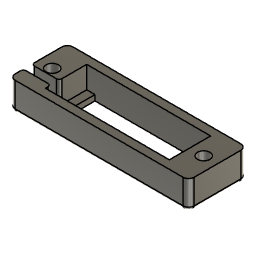
BracketLD2450 (Autodesk Fusion 360 design; units mm, degrees)
Autodesk Fusion 360 part; units mm, degrees
note: some values were not read from the file. Set by a fixed rule: the direction of a hole.
sketch "Sketch1" plane through (0, 0, 0) normal (0, 0, 1) x (1, 0, 0)
  line L0 (0, 0) -> (45, 0)
  line L1 (45, 0) -> (45, 15)
  line L2 (45, 15) -> (0, 15)
  line L3 (0, 15) -> (0, 0)
  line L4 (-10, -3) -> (55, -3)
  line L5 (55, -3) -> (55, 18)
  line L6 (55, 18) -> (-10, 18)
  line L7 (-10, 18) -> (-10, -3)
  line L8 (0, 7.5) -> (-5, 7.5)
  line L9 (45, 7.5) -> (50, 7.5)
  line L10 (0, 15) -> (3, 15)
  line L11 (3, 15) -> (3, 0)
  line L12 (3, 0) -> (0, 0)
  line L13 (0, 0) -> (0, 15)
  line L14 (45, 15) -> (42, 15)
  line L15 (42, 15) -> (42, 0)
  line L16 (42, 0) -> (45, 0)
  line L17 (45, 0) -> (45, 15)
  line L18 (0, 0) -> (0, 2)
  line L19 (0, 2) -> (-10, 2)
  line L20 (-10, 2) -> (-10, 5)
  line L21 (-10, 5) -> (0, 5)
  line L22 (0, 5) -> (0, 2)
  dimension "d1" = 45
  dimension "d2" = 15
  dimension "d5" = 65
  dimension "d6" = 21
  dimension "d7" = 5
  dimension "d8" = 5
  dimension "d9" = 3
  dimension "d10" = 15
  dimension "d11" = 3
  dimension "d19" = 2
  dimension "d20" = 3
  constraint horizontal L0
  constraint vertical L1
  constraint horizontal L2
  constraint vertical L3
  constraint coincident L0.start L3.end
  constraint horizontal L4
  constraint vertical L5
  constraint horizontal L6
  constraint vertical L7
  constraint midpoint L3 L8.start
  constraint perpendicular L7 L8
  constraint midpoint L1 L9.start
  constraint perpendicular L1 L9
  constraint horizontal L10
  constraint vertical L11
  constraint horizontal L12
  constraint vertical L13
  constraint horizontal L14
  constraint vertical L15
  constraint horizontal L16
  constraint vertical L17
  constraint perpendicular L12 L18
  constraint horizontal L19
  constraint vertical L20
  constraint horizontal L21
  constraint vertical L22
  measures "d1" distance of L0.start L0.end
  measures "d2" distance of L0.start L2.end
  measures "d5" distance of L4.start L4.end
  measures "d6" distance of L4.start L6.end
  measures "d7" distance of L8.start L8.end
  measures "d8" distance of L9.start L9.end
  measures "d9" distance of L2.end L10.end
  measures "d10" distance of L2.end L0.start
  measures "d11" distance of L1.end L14.end
  measures "d19" distance of L0.start L18.end
  measures "d20" distance of L18.end L21.end
extrude "Extrude1" add sketch "Sketch1" along normal blind 8 contours L0 L2 L3 L10 L11 L12 L13 L18 L22 | L0 L1 L2 L3 L4 L5 L6 L7 L10 L12 L13 L14 L16 L17 L18 L19 L21 | L3 L7 L13 L19 L20 L21 L22 | L0 L1 L2 L14 L15 L16 L17
extrude "Extrude2" cut sketch "Sketch1" along normal blind 100 from surface at 2 contours L0 L2 L3 L10 L11 L12 L13 L18 L22 | L0 L1 L2 L14 L15 L16 L17
extrude "Extrude3" add 1 faces at (-6.6667, 5, 8) along direction (0, 0, 1) blind 2
extrude "Extrude4" cut sketch "Sketch1" along normal blind 100 from surface at 3 contours L3 L7 L13 L19 L20 L21 L22
hole "Hole1" at (50, 7.5, 0) at (-5, 7.5, 0) direction (0, 0, 1) diameter 4.5 depth 20 tip angle 118
move_face "OffsetFaces1" offset -1 1 faces at (16, 15, 7.3333)
move_face "OffsetFaces2" offset -1 1 faces at (29, 0, 7.3333)
fillet "Fillet1" radius 1 4 edges at (22.5, 18, 0) (-10, 7.5, 0) (22.5, -3, 0) (55, 7.5, 0)
fillet "Fillet2" radius 2 8 edges at (-9.7071, 17.7071, 0.2929) (-10, 18, 5.5) (-9.7071, -2.7071, 0.2929) (-10, -3, 5.5) (54.7071, -2.7071, 0.2929) (55, -3, 5.5) (54.7071, 17.7071, 0.2929) (55, 18, 5.5)
fillet "Fillet3" radius 1 4 edges at (0, 2, 6.5) (-10, 2, 6.5) (0, 5, 6.5) (-10, 5, 6.5)
fillet "Fillet4" radius 1 1 edges at (0, 3.5, 3)
fillet "Fillet5" radius 1 1 edges at (-10, 3.5, 3)
move_face "OffsetFaces3" offset 1 1 faces at (16, 16, 7.3333)
move_face "OffsetFaces4" offset 1 1 faces at (29, -1, 7.3333)
equation "d5 = 20 mm + 45 mm"
equation "d6 = 6 mm + 15 mm"
